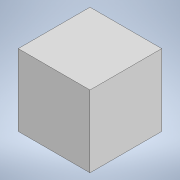
# Autodesk Inventor part: Extrusion1
Saved by Autodesk Inventor 2021 (Build 250183000, 183)
## iProperties
Created: 2022-12-02
Part Number: Extrusion1
Material: 常规
Document SubType Name: Modeling
Designer: skarn
Density: 1 g/cm^3
Appearance: 默认
Author: skarn
Autodesk Inventor part; units mm, degrees
ref_plane "YZ Plane" through (0, 0, 0) normal (1, 0, 0) x (0, 1, 0)
ref_plane "XZ Plane" through (0, 0, 0) normal (0, 1, 0) x (-1, 0, 0)
ref_plane "XY Plane" through (0, 0, 0) normal (0, 0, 1) x (1, 0, 0)
sketch "Sketch" plane through (0, 0, 0) normal (0, 0, 1) x (1, 0, 0)
  line L0 (0, 0) -> (500, 0)
  line L1 (500, 0) -> (500, 500)
  line L2 (500, 500) -> (0, 500)
  line L3 (0, 500) -> (0, 0)
  constraints: 8 end point, 2 parallel, 1 horizontal, 1 perpendicular
extrude "Extrusion" add sketch "Sketch" along normal mid plane 500
